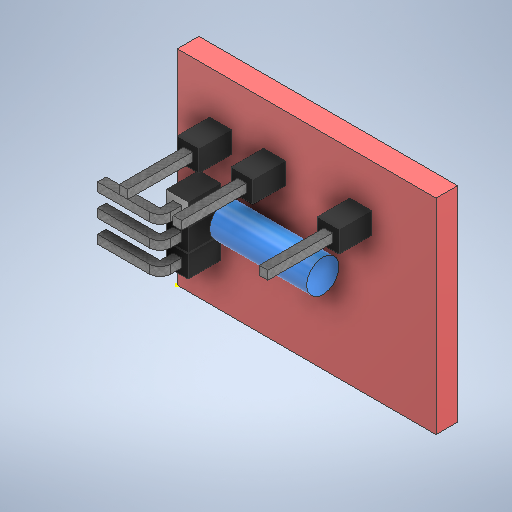
# Autodesk Inventor part: Circuit
Saved by Autodesk Inventor 2025.1 (Build 291241020, 241B)
## iProperties
Created: 2024-08-30
Part Number: Circuit
Material: Generic
Document SubType Name: Modeling
Designer: andre
Density: 1 g/cm^3
Appearance: Default
Author: andre
Autodesk Inventor part; units mm, degrees
ref_plane "YZ Plane" through (0, 0, 0) normal (1, 0, 0) x (0, 1, 0)
ref_plane "XZ Plane" through (0, 0, 0) normal (0, 1, 0) x (-1, 0, 0)
sketch "Sketch1" plane through (0, 0, 0) normal (0, 0, 1) x (1, 0, 0)
  line L0 (0, 0) -> (24, 0)
  line L1 (24, 0) -> (24, 19)
  line L2 (24, 19) -> (0, 19)
  line L3 (0, 19) -> (0, 0)
  dimension "d0" = 24
  dimension "d1" = 19
  constraints: 8 end point, 2 parallel, 1 horizontal, 1 perpendicular
  measures "d0" distance of L1.end L2.end
  measures "d1" distance of L0.end L1.end
extrude "Extrusion1" add sketch "Sketch1" along normal blind 2
ref_plane "Work Plane1" through (15, 0, 0) normal (1, 0, 0) x (0, 0, -1)
sketch "Sketch2" plane through (15, 0, 0) normal (1, 0, 0) x (0, 0, -1)
  circle A0 centre (-3.5, 9) radius 1.5
  line L0 (-2, 0) -> (-2, 19) projected
  line L1 (0, 0) -> (-2, 0) projected
  dimension "d5" = 3
  dimension "d6" = 9
  constraints: 1 centre point, 1 tangent
  measures "d5" diameter of A0
  measures "d6" distance from line of L1 A0.centre
extrude "Extrusion2" add sketch "Sketch2" against normal blind 9
sketch "Sketch3" plane through (0, 0, 2) normal (0, 0, 1) x (1, 0, 0)
  point P0 (0, 0)
sketch "Sketch4" plane through (0, 0, 2) normal (0, 0, 1) x (1, 0, 0)
  line L0 (3, 15) -> (5, 15)
  line L1 (5, 15) -> (5, 13)
  line L2 (5, 13) -> (3, 13)
  line L3 (3, 13) -> (3, 15)
  line L4 (2, 10.2) -> (4, 10.2)
  line L5 (4, 10.2) -> (4, 8.2)
  line L6 (4, 8.2) -> (2, 8.2)
  line L7 (2, 8.2) -> (2, 10.2)
  line L8 (2, 8.1) -> (4, 8.1)
  line L9 (4, 8.1) -> (4, 6.1)
  line L10 (4, 6.1) -> (2, 6.1)
  line L11 (2, 6.1) -> (2, 8.1)
  line L12 (2, 6) -> (4, 6)
  line L13 (4, 6) -> (4, 4)
  line L14 (4, 4) -> (2, 4)
  line L15 (2, 4) -> (2, 6)
  line L16 (16, 15) -> (18, 15)
  line L17 (18, 15) -> (18, 13)
  line L18 (18, 13) -> (16, 13)
  line L19 (16, 13) -> (16, 15)
  line L20 (8, 15) -> (10, 15)
  line L21 (10, 15) -> (10, 13)
  line L22 (10, 13) -> (8, 13)
  line L23 (8, 13) -> (8, 15)
  line L24 (24, 0) -> (24, 19) projected
  line L25 (24, 19) -> (0, 19) projected
  line L26 (0, 0) -> (24, 0) projected
  line L27 (0, 19) -> (0, 0) projected
  point P0 (5, 14)
  point P1 (3, 8.2)
  dimension "d9" = 2
  dimension "d10" = 2
  dimension "d11" = 2
  dimension "d12" = 2
  dimension "d13" = 2
  dimension "d14" = 2
  dimension "d15" = 2
  dimension "d16" = 2
  dimension "d17" = 2
  dimension "d18" = 2
  dimension "d19" = 2
  dimension "d20" = 2
  dimension "d21" = 6
  dimension "d22" = 14
  dimension "d23" = 19
  dimension "d24" = 4
  dimension "d25" = 4
  dimension "d26" = 0.1
  dimension "d27" = 0.1
  dimension "d28" = 2
  constraints: 48 end point, 12 parallel, 6 horizontal, 6 perpendicular, 2 horizontal alignment, 2 midpoint, 2 vertical alignment
  measures "d9" distance of L1.end L2.end
  measures "d10" distance of L0.end L1.end
  measures "d11" distance of L5.end L6.end
  measures "d12" distance of L4.end L5.end
  measures "d13" distance of L9.end L10.end
  measures "d14" distance of L8.end L9.end
  measures "d15" distance of L13.end L14.end
  measures "d16" distance of L12.end L13.end
  measures "d17" distance of L17.end L18.end
  measures "d18" distance of L16.end L17.end
  measures "d19" distance of L21.end L22.end
  measures "d20" distance of L20.end L21.end
  measures "d21" distance between parallel lines of L17 L24
  measures "d22" distance between parallel lines of L21 L24
  measures "d23" distance from line of point (5, 14) L24
  measures "d24" distance between parallel lines of L25 L0
  measures "d25" distance between parallel lines of L14 L26
  measures "d26" distance between parallel lines of L10 L12
  measures "d27" distance from line of point (3, 8.2) L8
  measures "d28" distance between parallel lines of L27 L7
extrude "Extrusion3" add sketch "Sketch4" along normal blind 3 contours L0 L1 L2 L3 | L4 L5 L6 L7 | L8 L9 L10 L11 | L12 L13 L14 L15 | L16 L17 L18 L19 | L20 L21 L22 L23
sketch "Sketch5" plane through (0, 0, 5) normal (0, 0, 1) x (1, 0, 0)
  line L0 (2, 8.2) -> (4, 8.2) projected
  line L1 (4, 8.2) -> (4, 10.2) projected
  line L2 (4, 10.2) -> (2, 10.2) projected
  line L3 (2, 10.2) -> (2, 8.2) projected
  line L4 (2, 6.1) -> (4, 6.1) projected
  line L5 (4, 6.1) -> (4, 8.1) projected
  line L6 (4, 8.1) -> (2, 8.1) projected
  line L7 (2, 8.1) -> (2, 6.1) projected
  line L8 (2, 4) -> (4, 4) projected
  line L9 (4, 4) -> (4, 6) projected
  line L10 (4, 6) -> (2, 6) projected
  line L11 (2, 6) -> (2, 4) projected
  line L12 (3, 13) -> (5, 13) projected
  line L13 (5, 13) -> (5, 15) projected
  line L14 (5, 15) -> (3, 15) projected
  line L15 (3, 15) -> (3, 13) projected
  line L16 (8, 13) -> (10, 13) projected
  line L17 (10, 13) -> (10, 15) projected
  line L18 (10, 15) -> (8, 15) projected
  line L19 (8, 15) -> (8, 13) projected
  line L20 (16, 13) -> (18, 13) projected
  line L21 (18, 13) -> (18, 15) projected
  line L22 (18, 15) -> (16, 15) projected
  line L23 (16, 15) -> (16, 13) projected
  line L24 (3.6, 14.4) -> (4.4, 14.4)
  line L25 (4.4, 14.4) -> (4.4, 13.6)
  line L26 (4.4, 13.6) -> (3.6, 13.6)
  line L27 (3.6, 13.6) -> (3.6, 14.4)
  line L28 (3, 15) -> (5, 13) construction
  line L29 (5, 15) -> (3, 15) construction
  line L30 (5, 15) -> (3, 13) construction
  line L31 (16.6, 14.4) -> (17.4, 14.4)
  line L32 (17.4, 14.4) -> (17.4, 13.6)
  line L33 (17.4, 13.6) -> (16.6, 13.6)
  line L34 (16.6, 13.6) -> (16.6, 14.4)
  line L35 (8.6, 14.4) -> (9.4, 14.4)
  line L36 (9.4, 14.4) -> (9.4, 13.6)
  line L37 (9.4, 13.6) -> (8.6, 13.6)
  line L38 (8.6, 13.6) -> (8.6, 14.4)
  line L39 (2.6, 9.6) -> (3.4, 9.6)
  line L40 (3.4, 9.6) -> (3.4, 8.8)
  line L41 (3.4, 8.8) -> (2.6, 8.8)
  line L42 (2.6, 8.8) -> (2.6, 9.6)
  line L43 (2.6, 5.4) -> (3.4, 5.4)
  line L44 (3.4, 5.4) -> (3.4, 4.6)
  line L45 (3.4, 4.6) -> (2.6, 4.6)
  line L46 (2.6, 4.6) -> (2.6, 5.4)
  line L47 (2.6, 7.5) -> (3.4, 7.5)
  line L48 (3.4, 7.5) -> (3.4, 6.7)
  line L49 (3.4, 6.7) -> (2.6, 6.7)
  line L50 (2.6, 6.7) -> (2.6, 7.5)
  point P0 (0, 0)
  point P1 (3.6, 14)
  point P2 (3, 14)
  point P3 (4, 14.4)
  point P4 (4, 14)
  point P5 (16.6, 14)
  point P6 (17, 14.4)
  point P7 (8.6, 14)
  point P8 (9, 14.4)
  point P9 (2.6, 9.2)
  point P10 (3, 9.6)
  point P11 (2.6, 5)
  point P12 (3, 5.4)
  point P13 (2.6, 7.1)
  point P14 (3, 7.5)
  point P15 (4.4, 14)
  point P16 (9, 15)
  point P17 (17, 15)
  point P18 (3, 10.2)
  point P19 (3, 8.1)
  point P20 (3, 6.1)
  point P21 (2, 9.2)
  point P22 (2, 7.1)
  point P23 (2, 5)
  dimension "d31" = 0.8
  dimension "d32" = 0.8
  dimension "d33" = 0.8
  dimension "d34" = 0.8
  dimension "d35" = 0.8
  dimension "d36" = 0.8
  dimension "d37" = 0.8
  dimension "d38" = 0.8
  dimension "d39" = 0.8
  dimension "d40" = 0.8
  dimension "d41" = 0.8
  dimension "d42" = 0.8
  constraints: 52 end point, 23 midpoint, 12 parallel, 7 perpendicular, 6 horizontal, 6 horizontal alignment, 6 vertical alignment
  measures "d31" distance of L24.start L24.end
  measures "d32" distance of L24.end L25.end
  measures "d33" distance of L31.start L31.end
  measures "d34" distance of L31.end L32.end
  measures "d35" distance of L35.start L35.end
  measures "d36" distance of L35.end L36.end
  measures "d37" distance of L39.start L39.end
  measures "d38" distance of L39.end L40.end
  measures "d39" distance of L43.start L43.end
  measures "d40" distance of L43.end L44.end
  measures "d41" distance of L47.start L47.end
  measures "d42" distance of L47.end L48.end
extrude "Extrusion4" add sketch "Sketch5" along normal blind 6 contours L24 L25 L26 L27 | L31 L32 L33 L34 | L35 L36 L37 L38
sketch "Sketch6" plane through (0, 0, 5) normal (0, 0, 1) x (1, 0, 0)
  line L0 (2, 8.2) -> (4, 8.2) projected
  line L1 (4, 8.2) -> (4, 10.2) projected
  line L2 (4, 10.2) -> (2, 10.2) projected
  line L3 (2, 10.2) -> (2, 8.2) projected
  line L4 (2, 6.1) -> (4, 6.1) projected
  line L5 (4, 6.1) -> (4, 8.1) projected
  line L6 (4, 8.1) -> (2, 8.1) projected
  line L7 (2, 8.1) -> (2, 6.1) projected
  line L8 (2, 4) -> (4, 4) projected
  line L9 (4, 4) -> (4, 6) projected
  line L10 (4, 6) -> (2, 6) projected
  line L11 (2, 6) -> (2, 4) projected
  line L12 (2.6, 9.6) -> (3.4, 9.6)
  line L13 (3.4, 9.6) -> (3.4, 8.8)
  line L14 (3.4, 8.8) -> (2.6, 8.8)
  line L15 (2.6, 8.8) -> (2.6, 9.6)
  line L16 (2.6, 7.5) -> (3.4, 7.5)
  line L17 (3.4, 7.5) -> (3.4, 6.7)
  line L18 (3.4, 6.7) -> (2.6, 6.7)
  line L19 (2.6, 6.7) -> (2.6, 7.5)
  line L20 (2.6, 5.4) -> (3.4, 5.4)
  line L21 (3.4, 5.4) -> (3.4, 4.6)
  line L22 (3.4, 4.6) -> (2.6, 4.6)
  line L23 (2.6, 4.6) -> (2.6, 5.4)
  line L24 (4, 10.2) -> (2, 10.2) projected
  point P0 (0, 0)
  point P1 (3, 7.5)
  point P2 (3, 10.2)
  point P3 (3, 5.4)
  point P4 (3, 10.2)
  point P5 (3, 9.6)
  point P6 (3, 6.1)
  point P7 (2.6, 9.2)
  point P8 (2, 9.2)
  point P9 (2.6, 7.1)
  point P10 (2, 7.1)
  point P11 (2.6, 5)
  point P12 (2, 5)
  dimension "d45" = 0.8
  dimension "d46" = 0.8
  dimension "d47" = 0.8
  dimension "d48" = 0.8
  dimension "d49" = 0.8
  dimension "d50" = 0.8
  constraints: 24 end point, 12 midpoint, 6 parallel, 3 horizontal, 3 horizontal alignment, 3 perpendicular, 3 vertical alignment
  measures "d45" distance of L13.end L14.end
  measures "d46" distance of L12.end L13.end
  measures "d47" distance of L18.start L18.end
  measures "d48" distance of L16.end L18.start
  measures "d49" distance of L22.start L22.end
  measures "d50" distance of L20.end L22.start
extrude "Extrusion5" add sketch "Sketch6" along normal blind 2 contours L12 L13 L14 L15 | L16 L17 L18 L19 | L20 L21 L22 L23
sketch "Sketch7" plane through (2.6, 8.8, 5) normal (-1, 0, 0) x (0, 0, 1)
  line L0 (0, 0) -> (0, 0.8) projected
  line L1 (0, 0) -> (2, 0) projected
  line L2 (2, 0.8) -> (2, 0) projected
  line L3 (0, 0.8) -> (2, 0.8) projected
  line L4 (0, -2.1) -> (0, -1.3) projected
  line L5 (0, -2.1) -> (2, -2.1) projected
  line L6 (2, -1.3) -> (2, -2.1) projected
  line L7 (0, -1.3) -> (2, -1.3) projected
  line L8 (0, -4.2) -> (0, -3.4) projected
  line L9 (0, -4.2) -> (2, -4.2) projected
  line L10 (2, -3.4) -> (2, -4.2) projected
  line L11 (0, -3.4) -> (2, -3.4) projected
  line L12 (2, 0.8) -> (1.2, 0.8)
  line L13 (1.2, 0.8) -> (1.2, 0)
  line L14 (1.2, 0) -> (2, 0)
  line L15 (2, 0) -> (2, 0.8)
  line L16 (2, -1.3) -> (1.2, -1.3)
  line L17 (1.2, -1.3) -> (1.2, -2.1)
  line L18 (1.2, -2.1) -> (2, -2.1)
  line L19 (2, -2.1) -> (2, -1.3)
  line L20 (2, -3.4) -> (1.2, -3.4)
  line L21 (1.2, -3.4) -> (1.2, -4.2)
  line L22 (1.2, -4.2) -> (2, -4.2)
  line L23 (2, -4.2) -> (2, -3.4)
  point P0 (-5, -8.8)
  point P1 (1.2, -3.4)
  point P2 (1.2, -1.3)
  point P3 (1.2, 0.8)
  dimension "d53" = 0.8
  dimension "d54" = 0.8
  dimension "d55" = 0.8
  constraints: 24 end point, 6 parallel, 3 horizontal, 3 perpendicular, 3 point on line
  measures "d53" distance of L14.end L13.end
  measures "d54" distance of L18.end L17.end
  measures "d55" distance of L22.end L21.end
extrude "Extrusion6" add sketch "Sketch7" along normal blind 5 contours L13 L3 L2 L1 | L17 L7 L6 L5 | L21 L11 L10 L9
fillet "Fillet1" radius 1 3 edges at (3.4, 9.2, 7) (3.4, 7.1, 7) (3.4, 5, 7)
sketch "Sketch8" plane through (0, 0, 0) normal (-1, 0, 0) x (0, 0, 1)
  line L0 (0, 19) -> (0, 0) projected
  line L1 (0, 0) -> (2, 0) projected
  line L2 (2, 19) -> (2, 0) projected
  line L3 (0, 19) -> (2, 19) projected
  line L4 (0, 0) -> (2, 19) construction
  line L5 (0, 19) -> (2, 0) construction
  line L6 (2, 6) -> (2, 4) construction
  line L7 (2, 10.2) -> (5, 10.2) construction
  line L8 (2, 4) -> (5, 10.2) construction
  line L9 (2, 10.2) -> (5, 4) construction
  point P0 (3.5, 7.1)
  point P1 (1, 9.5)
  dimension "d59" = 2.4
  constraints: 8 end point, 2 midpoint
  measures "d59" vertical distance of point (3.5, 7.1) point (1, 9.5)
body "Solid1"
